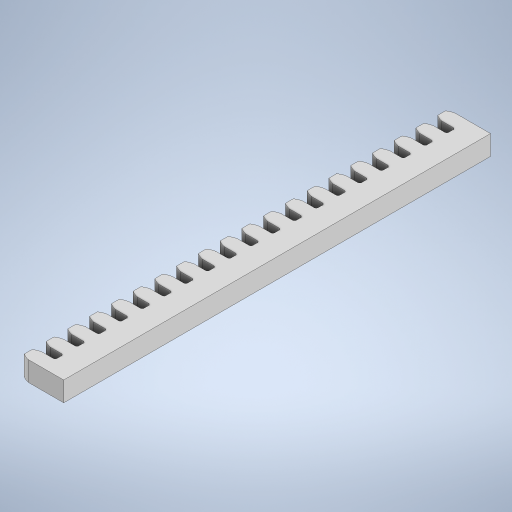
# Autodesk Inventor part: GearTrack
Saved by Autodesk Inventor 2024 (Build 280153000, 153)
## iProperties
Created: 2024-08-13
Part Number: GearTrack
Material: Generic
Document SubType Name: Modeling
Designer: eltic
Density: 1 g/cm^3
Appearance: Default
Author: eltic
Autodesk Inventor part; units mm, degrees
ref_plane "YZ Plane" through (0, 0, 0) normal (1, 0, 0) x (0, 1, 0)
ref_plane "XZ Plane" through (0, 0, 0) normal (0, 1, 0) x (-1, 0, 0)
ref_plane "XY Plane" through (0, 0, 0) normal (0, 0, 1) x (1, 0, 0)
sketch "Sketch3" plane through (0, 0, 0) normal (0, 1, 0) x (-1, 0, 0)
  line L0 (4.6541, 1.1087) -> (2.9213, 1.1087)
  arc A0 (2.6238, 1.3702) -> (2.9213, 1.1087) centre (2.9213, 1.4087) ccw
  arc A1 (5.6813, 0.6887) -> (4.6541, 1.1087) centre (4.052, -1.8303) ccw
  arc A2 (5.6813, -0.5113) -> (5.6813, 0.6887) centre (-8.3059, 0.0887) ccw
  arc A3 (4.6541, -0.9313) -> (5.6813, -0.5113) centre (4.052, 2.0077) ccw
  line L1 (4.6541, -0.9313) -> (2.9213, -0.9313)
  arc A4 (2.9213, -0.9313) -> (2.6238, -1.1928) centre (2.9213, -1.2313) ccw
  line L2 (-0.7132, 1.1087) -> (-0.7132, -63.6298)
  line L3 (-0.7132, -63.6298) -> (2.6238, -63.6298)
  line L4 (2.6238, -63.6298) -> (2.6238, 1.3702)
  arc A5 (2.9213, -4.2313) -> (2.6238, -4.4928) centre (2.9213, -4.5313) ccw
  line L5 (4.6541, -2.1913) -> (2.9213, -2.1913)
  line L6 (4.6541, -4.2313) -> (2.9213, -4.2313)
  arc A6 (5.6813, -2.6113) -> (4.6541, -2.1913) centre (4.052, -5.1303) ccw
  arc A7 (5.6813, -3.8113) -> (5.6813, -2.6113) centre (-8.3059, -3.2113) ccw
  arc A8 (4.6541, -4.2313) -> (5.6813, -3.8113) centre (4.052, -1.2923) ccw
  arc A9 (2.6238, -1.9298) -> (2.9213, -2.1913) centre (2.9213, -1.8913) ccw
  arc A10 (2.9213, -7.5313) -> (2.6238, -7.7928) centre (2.9213, -7.8313) ccw
  line L7 (4.6541, -5.4913) -> (2.9213, -5.4913)
  line L8 (4.6541, -7.5313) -> (2.9213, -7.5313)
  arc A11 (5.6813, -5.9113) -> (4.6541, -5.4913) centre (4.052, -8.4303) ccw
  arc A12 (5.6813, -7.1113) -> (5.6813, -5.9113) centre (-8.3059, -6.5113) ccw
  arc A13 (4.6541, -7.5313) -> (5.6813, -7.1113) centre (4.052, -4.5923) ccw
  arc A14 (2.6238, -5.2298) -> (2.9213, -5.4913) centre (2.9213, -5.1913) ccw
  arc A15 (2.9213, -10.8313) -> (2.6238, -11.0928) centre (2.9213, -11.1313) ccw
  line L9 (4.6541, -8.7913) -> (2.9213, -8.7913)
  line L10 (4.6541, -10.8313) -> (2.9213, -10.8313)
  arc A16 (5.6813, -9.2113) -> (4.6541, -8.7913) centre (4.052, -11.7303) ccw
  arc A17 (5.6813, -10.4113) -> (5.6813, -9.2113) centre (-8.3059, -9.8113) ccw
  arc A18 (4.6541, -10.8313) -> (5.6813, -10.4113) centre (4.052, -7.8923) ccw
  arc A19 (2.6238, -8.5298) -> (2.9213, -8.7913) centre (2.9213, -8.4913) ccw
  arc A20 (2.9213, -14.1313) -> (2.6238, -14.3928) centre (2.9213, -14.4313) ccw
  line L11 (4.6541, -12.0913) -> (2.9213, -12.0913)
  line L12 (4.6541, -14.1313) -> (2.9213, -14.1313)
  arc A21 (5.6813, -12.5113) -> (4.6541, -12.0913) centre (4.052, -15.0303) ccw
  arc A22 (5.6813, -13.7113) -> (5.6813, -12.5113) centre (-8.3059, -13.1113) ccw
  arc A23 (4.6541, -14.1313) -> (5.6813, -13.7113) centre (4.052, -11.1923) ccw
  arc A24 (2.6238, -11.8298) -> (2.9213, -12.0913) centre (2.9213, -11.7913) ccw
  arc A25 (2.9213, -17.4313) -> (2.6238, -17.6928) centre (2.9213, -17.7313) ccw
  line L13 (4.6541, -15.3913) -> (2.9213, -15.3913)
  line L14 (4.6541, -17.4313) -> (2.9213, -17.4313)
  arc A26 (5.6813, -15.8113) -> (4.6541, -15.3913) centre (4.052, -18.3303) ccw
  arc A27 (5.6813, -17.0113) -> (5.6813, -15.8113) centre (-8.3059, -16.4113) ccw
  arc A28 (4.6541, -17.4313) -> (5.6813, -17.0113) centre (4.052, -14.4923) ccw
  arc A29 (2.6238, -15.1298) -> (2.9213, -15.3913) centre (2.9213, -15.0913) ccw
  arc A30 (2.9213, -20.7313) -> (2.6238, -20.9928) centre (2.9213, -21.0313) ccw
  line L15 (4.6541, -18.6913) -> (2.9213, -18.6913)
  line L16 (4.6541, -20.7313) -> (2.9213, -20.7313)
  arc A31 (5.6813, -19.1113) -> (4.6541, -18.6913) centre (4.052, -21.6303) ccw
  arc A32 (5.6813, -20.3113) -> (5.6813, -19.1113) centre (-8.3059, -19.7113) ccw
  arc A33 (4.6541, -20.7313) -> (5.6813, -20.3113) centre (4.052, -17.7923) ccw
  arc A34 (2.6238, -18.4298) -> (2.9213, -18.6913) centre (2.9213, -18.3913) ccw
  arc A35 (2.9213, -24.0313) -> (2.6238, -24.2928) centre (2.9213, -24.3313) ccw
  line L17 (4.6541, -21.9913) -> (2.9213, -21.9913)
  line L18 (4.6541, -24.0313) -> (2.9213, -24.0313)
  arc A36 (5.6813, -22.4113) -> (4.6541, -21.9913) centre (4.052, -24.9303) ccw
  arc A37 (5.6813, -23.6113) -> (5.6813, -22.4113) centre (-8.3059, -23.0113) ccw
  arc A38 (4.6541, -24.0313) -> (5.6813, -23.6113) centre (4.052, -21.0923) ccw
  arc A39 (2.6238, -21.7298) -> (2.9213, -21.9913) centre (2.9213, -21.6913) ccw
  arc A40 (2.9213, -27.3313) -> (2.6238, -27.5928) centre (2.9213, -27.6313) ccw
  line L19 (4.6541, -25.2913) -> (2.9213, -25.2913)
  line L20 (4.6541, -27.3313) -> (2.9213, -27.3313)
  arc A41 (5.6813, -25.7113) -> (4.6541, -25.2913) centre (4.052, -28.2303) ccw
  arc A42 (5.6813, -26.9113) -> (5.6813, -25.7113) centre (-8.3059, -26.3113) ccw
  arc A43 (4.6541, -27.3313) -> (5.6813, -26.9113) centre (4.052, -24.3923) ccw
  arc A44 (2.6238, -25.0298) -> (2.9213, -25.2913) centre (2.9213, -24.9913) ccw
  arc A45 (2.9213, -30.6313) -> (2.6238, -30.8928) centre (2.9213, -30.9313) ccw
  line L21 (4.6541, -28.5913) -> (2.9213, -28.5913)
  line L22 (4.6541, -30.6313) -> (2.9213, -30.6313)
  arc A46 (5.6813, -29.0113) -> (4.6541, -28.5913) centre (4.052, -31.5303) ccw
  arc A47 (5.6813, -30.2113) -> (5.6813, -29.0113) centre (-8.3059, -29.6113) ccw
  arc A48 (4.6541, -30.6313) -> (5.6813, -30.2113) centre (4.052, -27.6923) ccw
  arc A49 (2.6238, -28.3298) -> (2.9213, -28.5913) centre (2.9213, -28.2913) ccw
  arc A50 (2.9213, -33.9313) -> (2.6238, -34.1928) centre (2.9213, -34.2313) ccw
  line L23 (4.6541, -31.8913) -> (2.9213, -31.8913)
  line L24 (4.6541, -33.9313) -> (2.9213, -33.9313)
  arc A51 (5.6813, -32.3113) -> (4.6541, -31.8913) centre (4.052, -34.8303) ccw
  arc A52 (5.6813, -33.5113) -> (5.6813, -32.3113) centre (-8.3059, -32.9113) ccw
  arc A53 (4.6541, -33.9313) -> (5.6813, -33.5113) centre (4.052, -30.9923) ccw
  arc A54 (2.6238, -31.6298) -> (2.9213, -31.8913) centre (2.9213, -31.5913) ccw
  arc A55 (2.9213, -37.2313) -> (2.6238, -37.4928) centre (2.9213, -37.5313) ccw
  line L25 (4.6541, -35.1913) -> (2.9213, -35.1913)
  line L26 (4.6541, -37.2313) -> (2.9213, -37.2313)
  arc A56 (5.6813, -35.6113) -> (4.6541, -35.1913) centre (4.052, -38.1303) ccw
  arc A57 (5.6813, -36.8113) -> (5.6813, -35.6113) centre (-8.3059, -36.2113) ccw
  arc A58 (4.6541, -37.2313) -> (5.6813, -36.8113) centre (4.052, -34.2923) ccw
  arc A59 (2.6238, -34.9298) -> (2.9213, -35.1913) centre (2.9213, -34.8913) ccw
  arc A60 (2.9213, -40.5313) -> (2.6238, -40.7928) centre (2.9213, -40.8313) ccw
  line L27 (4.6541, -38.4913) -> (2.9213, -38.4913)
  line L28 (4.6541, -40.5313) -> (2.9213, -40.5313)
  arc A61 (5.6813, -38.9113) -> (4.6541, -38.4913) centre (4.052, -41.4303) ccw
  arc A62 (5.6813, -40.1113) -> (5.6813, -38.9113) centre (-8.3059, -39.5113) ccw
  arc A63 (4.6541, -40.5313) -> (5.6813, -40.1113) centre (4.052, -37.5923) ccw
  arc A64 (2.6238, -38.2298) -> (2.9213, -38.4913) centre (2.9213, -38.1913) ccw
  arc A65 (2.9213, -43.8313) -> (2.6238, -44.0928) centre (2.9213, -44.1313) ccw
  line L29 (4.6541, -41.7913) -> (2.9213, -41.7913)
  line L30 (4.6541, -43.8313) -> (2.9213, -43.8313)
  arc A66 (5.6813, -42.2113) -> (4.6541, -41.7913) centre (4.052, -44.7303) ccw
  arc A67 (5.6813, -43.4113) -> (5.6813, -42.2113) centre (-8.3059, -42.8113) ccw
  arc A68 (4.6541, -43.8313) -> (5.6813, -43.4113) centre (4.052, -40.8923) ccw
  arc A69 (2.6238, -41.5298) -> (2.9213, -41.7913) centre (2.9213, -41.4913) ccw
  arc A70 (2.9213, -47.1313) -> (2.6238, -47.3928) centre (2.9213, -47.4313) ccw
  line L31 (4.6541, -45.0913) -> (2.9213, -45.0913)
  line L32 (4.6541, -47.1313) -> (2.9213, -47.1313)
  arc A71 (5.6813, -45.5113) -> (4.6541, -45.0913) centre (4.052, -48.0303) ccw
  arc A72 (5.6813, -46.7113) -> (5.6813, -45.5113) centre (-8.3059, -46.1113) ccw
  arc A73 (4.6541, -47.1313) -> (5.6813, -46.7113) centre (4.052, -44.1923) ccw
  arc A74 (2.6238, -44.8298) -> (2.9213, -45.0913) centre (2.9213, -44.7913) ccw
  arc A75 (2.9213, -50.4313) -> (2.6238, -50.6928) centre (2.9213, -50.7313) ccw
  line L33 (4.6541, -48.3913) -> (2.9213, -48.3913)
  line L34 (4.6541, -50.4313) -> (2.9213, -50.4313)
  arc A76 (5.6813, -48.8113) -> (4.6541, -48.3913) centre (4.052, -51.3303) ccw
  arc A77 (5.6813, -50.0113) -> (5.6813, -48.8113) centre (-8.3059, -49.4113) ccw
  arc A78 (4.6541, -50.4313) -> (5.6813, -50.0113) centre (4.052, -47.4923) ccw
  arc A79 (2.6238, -48.1298) -> (2.9213, -48.3913) centre (2.9213, -48.0913) ccw
  arc A80 (2.9213, -53.7313) -> (2.6238, -53.9928) centre (2.9213, -54.0313) ccw
  line L35 (4.6541, -51.6913) -> (2.9213, -51.6913)
  line L36 (4.6541, -53.7313) -> (2.9213, -53.7313)
  arc A81 (5.6813, -52.1113) -> (4.6541, -51.6913) centre (4.052, -54.6303) ccw
  arc A82 (5.6813, -53.3113) -> (5.6813, -52.1113) centre (-8.3059, -52.7113) ccw
  arc A83 (4.6541, -53.7313) -> (5.6813, -53.3113) centre (4.052, -50.7923) ccw
  arc A84 (2.6238, -51.4298) -> (2.9213, -51.6913) centre (2.9213, -51.3913) ccw
  arc A85 (2.9213, -57.0313) -> (2.6238, -57.2928) centre (2.9213, -57.3313) ccw
  line L37 (4.6541, -54.9913) -> (2.9213, -54.9913)
  line L38 (4.6541, -57.0313) -> (2.9213, -57.0313)
  arc A86 (5.6813, -55.4113) -> (4.6541, -54.9913) centre (4.052, -57.9303) ccw
  arc A87 (5.6813, -56.6113) -> (5.6813, -55.4113) centre (-8.3059, -56.0113) ccw
  arc A88 (4.6541, -57.0313) -> (5.6813, -56.6113) centre (4.052, -54.0923) ccw
  arc A89 (2.6238, -54.7298) -> (2.9213, -54.9913) centre (2.9213, -54.6913) ccw
  arc A90 (2.9213, -60.3313) -> (2.6238, -60.5928) centre (2.9213, -60.6313) ccw
  line L39 (4.6541, -58.2913) -> (2.9213, -58.2913)
  line L40 (4.6541, -60.3313) -> (2.9213, -60.3313)
  arc A91 (5.6813, -58.7113) -> (4.6541, -58.2913) centre (4.052, -61.2303) ccw
  arc A92 (5.6813, -59.9113) -> (5.6813, -58.7113) centre (-8.3059, -59.3113) ccw
  arc A93 (4.6541, -60.3313) -> (5.6813, -59.9113) centre (4.052, -57.3923) ccw
  arc A94 (2.6238, -58.0298) -> (2.9213, -58.2913) centre (2.9213, -57.9913) ccw
  arc A95 (2.9213, -63.6313) -> (2.6238, -63.8928) centre (2.9213, -63.9313) ccw
  line L41 (4.6541, -61.5913) -> (2.9213, -61.5913)
  line L42 (4.6541, -63.6313) -> (2.9213, -63.6313)
  arc A96 (5.6813, -62.0113) -> (4.6541, -61.5913) centre (4.052, -64.5303) ccw
  arc A97 (5.6813, -63.2113) -> (5.6813, -62.0113) centre (-8.3059, -62.6113) ccw
  arc A98 (4.6541, -63.6313) -> (5.6813, -63.2113) centre (4.052, -60.6923) ccw
  arc A99 (2.6238, -61.3298) -> (2.9213, -61.5913) centre (2.9213, -61.2913) ccw
  line L43 (2.6238, -63.6298) -> (3.4498, -63.6313)
  line L44 (4.6541, 1.1087) -> (-0.7132, 1.1087)
  point P0 (0, 0)
  point P1 (5.6941, 0.0887)
  point P2 (5.6941, -3.2113)
  point P3 (5.6941, -6.5113)
  point P4 (5.6941, -9.8113)
  point P5 (5.6941, -13.1113)
  point P6 (5.6941, -16.4113)
  point P7 (5.6941, -19.7113)
  point P8 (5.6941, -23.0113)
  point P9 (5.6941, -26.3113)
  point P10 (5.6941, -29.6113)
  point P11 (5.6941, -32.9113)
  point P12 (5.6941, -36.2113)
  point P13 (5.6941, -39.5113)
  point P14 (5.6941, -42.8113)
  point P15 (5.6941, -46.1113)
  point P16 (5.6941, -49.4113)
  point P17 (5.6941, -52.7113)
  point P18 (5.6941, -56.0113)
  point P19 (5.6941, -59.3113)
  point P20 (5.6941, -62.6113)
  point P21 (2.6238, -61.3298)
  point P22 (2.6238, -60.5928)
  point P23 (2.6238, -58.0298)
  point P24 (2.6238, -57.2928)
  point P25 (2.6238, -54.7298)
  point P26 (2.6238, -53.9928)
  point P27 (2.6238, -51.4298)
  point P28 (2.6238, -50.6928)
  point P29 (2.6238, -48.1298)
  point P30 (2.6238, -47.3928)
  point P31 (2.6238, -44.8298)
  point P32 (2.6238, -44.0928)
  point P33 (2.6238, -41.5298)
  point P34 (2.6238, -40.7928)
  point P35 (2.6238, -37.4928)
  point P36 (2.6238, -34.1928)
  point P37 (2.6238, -30.8928)
  point P38 (2.6238, -27.5928)
  point P39 (2.6238, -24.2928)
  point P40 (2.6238, -20.9928)
  point P41 (2.6238, -18.4298)
  point P42 (2.6238, -17.6928)
  point P43 (2.6238, -15.1298)
  point P44 (2.6238, -14.3928)
  point P45 (2.6238, -11.8298)
  point P46 (2.6238, -11.0928)
  point P47 (2.6238, -8.5298)
  point P48 (2.6238, -7.7928)
  point P49 (2.6238, -5.2298)
  point P50 (2.6238, -4.4928)
  point P51 (2.6238, -1.9298)
  point P52 (2.6238, -1.1928)
  dimension "d16" = 0.6
  dimension "d17" = 1.2
  dimension "d18" = 3
  dimension "d19" = 3
  dimension "d21" = 65
  dimension "d25" = 3.3
  constraints: 266 vertical alignment, 201 point on circle, 100 centre point, 96 equal radius, 88 end point, 38 parallel, 2 horizontal, 2 tangent, 1 perpendicular, 1 point on line, 1 vertical, 3 other
  measures "d16" vertical distance of A2.start point (5.694, 0.089)
  measures "d17" distance of A1.start A2.start
  measures "d18" radius of A3
  measures "d19" radius of A1
  measures "d21" distance of L3.end A0.start
  measures "d25" distance of L1.end L6.end
extrude "Extrusion1" add sketch "Sketch3" along normal blind 3 contours A1 A2 A3 L1 A4 L4 L44 L0 | L4 L3 L2 L44 | A9 L5 A6 A7 A8 L6 A5 L4 | L4 A99 L41 A96 A97 A98 L42 L43 | A14 L7 A11 A12 A13 L8 A10 L4 | L4 A94 L39 A91 A92 A93 L40 A90 | A19 L9 A16 A17 A18 L10 A15 L4 | L4 A89 L37 A86 A87 A88 L38 A85 | A24 L11 A21 A22 A23 L12 A20 L4 | L4 A84 L35 A81 A82 A83 L36 A80 | A29 L13 A26 A27 A28 L14 A25 L4 | L4 A79 L33 A76 A77 A78 L34 A75 | A34 L15 A31 A32 A33 L16 A30 L4 | L4 A74 L31 A71 A72 A73 L32 A70 | A39 L17 A36 A37 A38 L18 A35 L4 | L4 A69 L29 A66 A67 A68 L30 A65 | A44 L19 A41 A42 A43 L20 A40 L4 | L4 A64 L27 A61 A62 A63 L28 A60 | A49 L21 A46 A47 A48 L22 A45 L4 | L4 A59 L25 A56 A57 A58 L26 A55 | A54 L23 A51 A52 A53 L24 A50 L4
body "Solid1"
